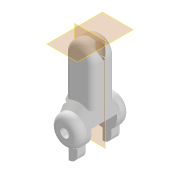
# Autodesk Inventor part: middle_f3
Saved by Autodesk Inventor 2020.2 (Build 242310000, 310)
## iProperties
Created: 2020-04-08
Part Number: middle_f3
Material: Generic
Document SubType Name: Modeling
Designer: Bardo91
Density: 1 g/cm^3
Appearance: Default
Author: Bardo91
Autodesk Inventor part; units mm, degrees
ref_plane "YZ Plane" through (0, 0, 0) normal (1, 0, 0) x (0, 1, 0)
ref_plane "XY Plane" through (0, 0, 0) normal (0, 0, 1) x (1, 0, 0)
sketch "Sketch1" plane through (0, 0, 0) normal (0, 0, 1) x (1, 0, 0)
  circle A0 centre (0, 0) radius 1.5
  circle A1 centre (0, 0) radius 5
  line L0 (0, 0) -> (0, 20)
  circle A2 centre (0, 20) radius 1.5
  circle A3 centre (0, 20) radius 5
  line L1 (-5, 20) -> (-5, 0)
  line L2 (5, 0) -> (5, 20)
  dimension "d0" = 3
  dimension "d1" = 10
  dimension "d2" = 20
  dimension "d3" = 3
  dimension "d4" = 10
  constraints: 6 end point, 4 centre point, 4 coincident, 4 point on circle, 3 tangent, 1 vertical
  measures "d0" diameter of A0
  measures "d1" diameter of A1
  measures "d2" distance of L0.start L0.end
  measures "d3" diameter of A2
  measures "d4" diameter of A3
extrude "base" add sketch "Sketch1" along normal blind 8 contours A1 | L1 A3 L0 A1 | A1 L0 A3 L2 | A3 | A2
sketch "Sketch2" plane through (0, 0, 8) normal (0, 0, 1) x (1, 0, 0)
  circle A0 centre (0, 0) radius 1.5
  circle A1 centre (0, 0) radius 5
  dimension "d7" = 3
  dimension "d8" = 10
  constraints: 2 centre point, 2 coincident
  measures "d7" diameter of A0
  measures "d8" diameter of A1
extrude "joint" add sketch "Sketch2" along normal blind 5
ref_plane "Work Plane1" through (0, 0, 4) normal (0, 0, 1) x (1, 0, 0)
mirror "Mirror1" about plane through (0, 0, 4) normal (0, 0, 1) of "joint"
chamfer "Chamfer1" distance 2 angle 45 2 edges at (0, 5, 0) (0, 5, 8)
fillet "Fillet1" radius 2 8 edges at (-5, 0, 13) (0, 25, 8) (-5, 12.4495, 8) (5, 12.4495, 8) (0, 25, 0) (-5, 12.4495, 0) (5, 12.4495, 0) (-5, 0, -5)
sketch "Sketch3" plane through (0, 0, 4) normal (0, 0, 1) x (1, 0, 0)
  circle A0 centre (0, 0) radius 5.25
  line L0 (0, 0) -> (-10, 0)
  line L1 (-10, 0) -> (-10, 5.25)
  line L2 (-10, 5.25) -> (0, 5.25)
  line L3 (0, 0) -> (0, 5.25)
  point P0 (-5.25, 0)
  dimension "d15" = 10.5
  dimension "d21" = 10
  dimension "d22" = 5.25
  constraints: 8 end point, 2 horizontal, 2 perpendicular, 1 coincident, 3 other
  measures "d21" distance of L0.start L0.end
  measures "d22" distance of L0.end L1.end
extrude "joint_2" cut sketch "Sketch3" along normal mid plane 9
sketch "Sketch9" plane through (0, 0, 0) normal (0, 1, 0) x (-1, 0, 0)
  line L0 (0, -0.5) -> (0, 8.5) projected
  line L1 (0, 4) -> (-3.5, 4)
  line L2 (0, 4) -> (3.5, 4)
  circle A0 centre (3.5, 4) radius 1.25
  circle A1 centre (-3.5, 4) radius 1.25
  point P0 (0, 0)
  dimension "d42" = 3.5
  dimension "d43" = 3.5
  dimension "d44" = 2.5
  dimension "thread_hole" = 2.5
  constraints: 4 end point, 2 centre point, 2 coincident, 2 horizontal, 1 midpoint
  measures "d42" distance of L1.start L1.end
  measures "d43" distance of L1.start L2.end
  measures "d44" diameter of A0
  measures "thread_hole" diameter of A1
extrude "thread_hole" cut sketch "Sketch9" along normal through all contours A1
sketch "Sketch10" plane through (0, 0, 8.5) normal (0, 0, -1) x (-1, 0, 0)
  line L0 (0, 0) -> (0, -6)
  line L1 (0, -6) -> (0, -9)
  line L2 (0, -9) -> (-3, -9)
  line L3 (-3, -9) -> (-3, -4)
  circle A0 centre (0, 0) radius 5 projected
  point P0 (0, -5)
  dimension "d48" = 6
  dimension "d49" = 3
  dimension "d50" = 3
  constraints: 8 end point, 1 horizontal, 1 perpendicular, 1 point on line, 1 vertical, 2 other
  measures "d48" distance of L0.start L0.end
  measures "d49" distance of L0.end L1.end
  measures "d50" distance of L1.end L2.end
extrude "lock" add sketch "Sketch10" against normal blind 3 contours L0 L1 L2 L3 A0
mirror "Mirror2" about plane through (0, 0, 4) normal (0, 0, 1) of "lock"
fillet "Fillet2" radius 3 2 edges at (3, -9, -2) (3, -9, 10)
sketch "Sketch11" plane through (0, 0, 4) normal (0, 0, 1) x (1, 0, 0)
  line L0 (-5, 20) -> (-5, 7.4833) projected
  line L1 (-5, 10.4833) -> (-1.5, 16.5455)
  point P0 (0, 0)
  dimension "d54" = 3
  dimension "d55" = 7
  constraints: 2 end point, 1 point on line
  measures "d54" distance of L0.end L1.start
  measures "d55" distance of L1.start L1.end
sketch "Sketch12" plane through (-5, 7.4833, 6) normal (-1, 0, 0) x (0, 0, 1)
  line L0 (0, 0) -> (0, 12.5167) projected
  line L1 (0, 0) -> (0, 3)
  line L2 (0, 3) -> (-2, 3)
  circle A0 centre (-2, 3) radius 1.25
  point P0 (-6, -7.4833)
  dimension "d57" = 3
  dimension "d58" = 2
  dimension "d59" = 2.5
  constraints: 4 end point, 1 centre point, 1 coincident, 1 perpendicular, 1 point on line
  measures "d57" distance of L0.start L1.end
  measures "d58" distance of L1.end L2.end
  measures "d59" diameter of A0
sweep "Sweep2" cut profiles "Sketch12" path "Sketch11" path curves L1
sketch "Sketch13" plane through (0, 0, 4) normal (0, 0, 1) x (1, 0, 0)
  line L0 (-1.5, 15.2955) -> (-1.5, 17.7955) projected
  circle A0 centre (-1.5, 16.5455) radius 1.25
  line L1 (-1.5, 15.2955) -> (-5, 15.2955)
  line L2 (-5, 7.4833) -> (-5, 20) projected
  line L3 (-1.5, 17.7955) -> (-5, 17.7955)
  line L4 (-5, 17.7955) -> (-5, 15.2955)
  point P0 (0, 0)
  constraints: 6 end point, 2 horizontal, 1 collinear, 1 midpoint, 1 parallel, 1 point on line, 3 other
extrude "Extrusion8" cut sketch "Sketch13" against normal mid plane 4
ref_plane "Work Plane3" through (0, 25, 0) normal (0, 1, 0) x (-1, 0, 0)
sketch "Sketch14" plane through (0, 25, 0) normal (0, 1, 0) x (-1, 0, 0)
  line L0 (0, -0.5) -> (0, 8.5) projected
  line L1 (0, 4) -> (-3.5, 4)
  circle A0 centre (-3.5, 4) radius 1.5
  point P0 (0, 0)
  dimension "d64" = 3.5
  dimension "d65" = 3
  constraints: 2 end point, 1 centre point, 1 coincident, 1 horizontal, 1 midpoint
  measures "d64" distance of L1.start L1.end
  measures "d65" diameter of A0
extrude "Extrusion9" cut sketch "Sketch14" against normal blind 5
equation "\"d44\" = thread_hole"
body "Solid1"
